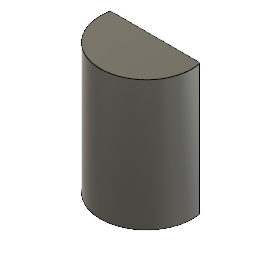
base_stepper_pin v2 (Autodesk Fusion 360 design; units mm, degrees)
Autodesk Fusion 360 part; units mm, degrees
sketch "Sketch1" plane through (0, 0, 0) normal (0, 1, 0) x (1, 0, 0)
  line L0 (0, 0) -> (0, 0.5)
  line L1 (0, 0.5) -> (0.1389, 0.5)
  line L2 (0.1389, 0.5) -> (2.424, 0.5)
  line L3 (0, 0.5) -> (-2.424, 0.5)
  arc A0 (-2.424, 0.5) -> (2.424, 0.5) centre (0, 0) ccw
  dimension "d1" = 4.95
  dimension "d2" = 0.5
  measures "d1" diameter of A0
extrude "Extrude1" add sketch "Sketch1" along normal blind 3
fillet "Fillet1" radius 0.1 2 edges at (2.424, 1.5, -0.5) (-2.424, 1.5, -0.5)
extrude "Extrude2" add 1 faces at (0, 3, 0.4917) along direction (0, 1, 0) blind 4
